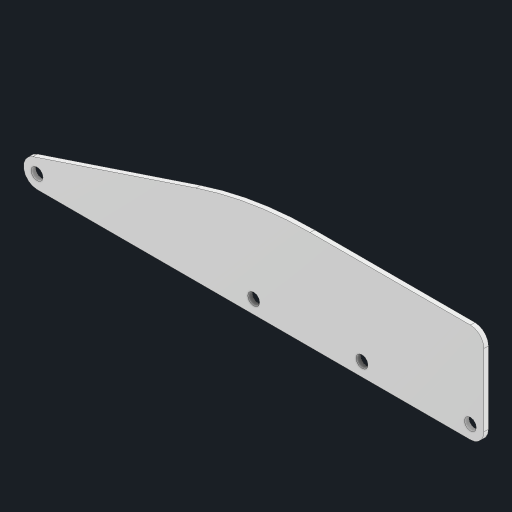
# Autodesk Inventor part: intake_base
Saved by Autodesk Inventor 2024 (Build 280153000, 153)
## iProperties
Created: 2023-08-21
Part Number: intake_base
Material: Acetal Resin, White
Document SubType Name: Modeling
Designer: Averey
Density: 1.425 g/cm^3
Appearance: Smooth - White
Author: Averey
Autodesk Inventor part; units mm, degrees
ref_plane "YZ Plane" through (0, 0, 0) normal (1, 0, 0) x (0, 1, 0)
ref_plane "XZ Plane" through (0, 0, 0) normal (0, 1, 0) x (-1, 0, 0)
ref_plane "XY Plane" through (0, 0, 0) normal (0, 0, 1) x (1, 0, 0)
sketch "Sketch1" plane through (0, 0, 0) normal (0, 0, 1) x (1, 0, 0)
  circle A0 centre (0, 0) radius 2.0955
  arc A1 (38.1, -4.7625) -> (42.8625, 0) centre (38.1, 0) ccw
  circle A2 centre (-38.1, 0) radius 2.0955
  circle A3 centre (38.1, 0) radius 2.0955
  circle A4 centre (-114.3, 0) radius 2.0955
  arc A5 (-115.806, 4.5181) -> (-114.3, -4.7625) centre (-114.3, 0) ccw
  arc A6 (42.8625, 25.4) -> (38.1, 30.1625) centre (38.1, 25.4) ccw
  line L0 (-115.806, 4.5181) -> (-58.4245, 23.6453)
  line L1 (-18.2636, 30.1625) -> (38.1, 30.1625)
  line L2 (42.8625, 25.4) -> (42.8625, 0)
  line L3 (38.1, -4.7625) -> (-114.3, -4.7625)
  line L4 (-39.606, 29.9181) -> (-38.8728, 30.1625)
  line L5 (-38.1, 30.1625) -> (-38.8728, 30.1625)
  arc A7 (-18.2636, 30.1625) -> (-58.4245, 23.6453) centre (-18.2636, -96.8375) ccw
  point P0 (0, 0)
  dimension "d1" = 38.1
  dimension "d3" = 4.191
  dimension "d4" = 4.191
  dimension "d5" = 4.191
  dimension "d8" = 9.525
  dimension "d11" = 127
  constraints: 12 end point, 8 centre point, 8 point on circle, 6 tangent, 3 coincident, 2 point on line, 1 horizontal, 1 horizontal alignment, 1 perpendicular, 2 other
  measures "d1" distance of A1.centre A0.centre
  measures "d3" diameter of A2
  measures "d4" diameter of A3
  measures "d5" diameter of A0
  measures "d8" diameter of A5
  measures "d11" radius of A7
extrude "Extrusion1" add sketch "Sketch1" along normal blind 1.5875
body "Solid1"
